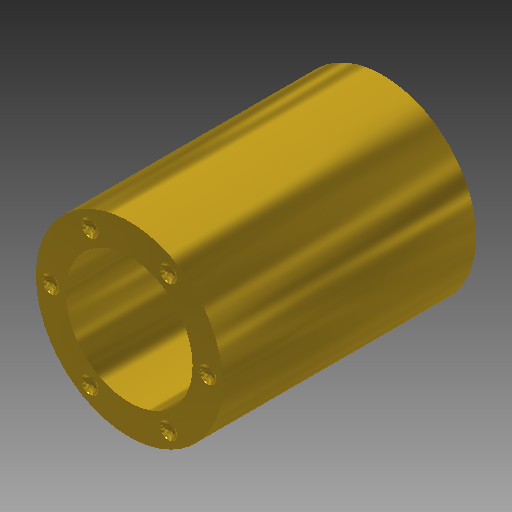
# Autodesk Inventor part: Electrode 1
Saved by Autodesk Inventor 2017 (Build 210142000, 142)
## iProperties
Created: 2009-05-06
Part Number: Electrode 1
Document SubType Name: Modeling
Designer: Serena
Material: Generic
Density: 1 g/cm^3
Appearance: Glossy - Gold
Author: Serena
Autodesk Inventor part; units mm, degrees
ref_plane "YZ Plane" through (0, 0, 0) normal (1, 0, 0) x (0, 1, 0)
ref_plane "XZ Plane" through (0, 0, 0) normal (0, 1, 0) x (-1, 0, 0)
ref_plane "XY Plane" through (0, 0, 0) normal (0, 0, 1) x (1, 0, 0)
sketch "Sketch1" plane through (0, 0, 0) normal (0, 0, 1) x (1, 0, 0)
  circle A0 centre (0, 0) radius 6.35
  circle A1 centre (0, 0) radius 9.35
  dimension "d0" = 12.7
  dimension "d1" = 18.7
  constraints: 2 centre point, 1 coincident
  measures "d0" diameter of A0
  measures "d1" diameter of A1
extrude "Extrusion1" add sketch "Sketch1" along normal blind 25.4
sketch "Sketch2" plane through (0, 0, 0) normal (0, 1, 0) x (-1, 0, 0)
  line L0 (-9.35, 0) -> (9.35, 0)
  line L1 (-9.35, 25.4) -> (9.35, 25.4)
  line L2 (-9.35, 25.4) -> (9.35, 25.4)
  line L3 (-9.35, 0) -> (9.35, 0)
  line L4 (6.35, 0) -> (6.35, 25.4)
  line L5 (9.35, 0) -> (9.35, 25.4)
  line L6 (-9.35, 0) -> (-9.35, 25.4)
  line L7 (-6.35, 0) -> (-6.35, 25.4)
  line L8 (7.85, 25.4) -> (7.85, 0)
  line L9 (7.85, 23.328674) -> (6.35, 23.328674)
  line L10 (9.35, 22.247069) -> (7.85, 22.247069)
  line L11 (12.106354, 26.15) -> (-10.018865, 26.15)
  line L12 (7.85, 25.4) -> (7.85, 27.239853)
  circle A0 centre (7.85, 26.15) radius 1
  line L13 (8.511438, 25.4) -> (7.188562, 25.4)
  line L14 (7.85, 25.4) -> (7.188562, 25.4)
  line L15 (7.85, 25.4) -> (7.85, 25.15)
  arc A1 (7.188562, 25.4) -> (7.85, 25.15) centre (7.85, 26.15) ccw
  dimension "d4" = 2
  dimension "d5" = 1.5
  constraints: 16 end point, 11 point on line, 5 point on circle, 4 perpendicular, 2 centre point, 2 concentric, 2 parallel, 1 collinear
  measures "d4" diameter of A0
  measures "d5" diameter of L1 L11
sketch "Sketch4" plane through (0, 0, 0) normal (0, 1, 0) x (-1, 0, 0)
  line L0 (9.35, 0) -> (9.35, 25.4)
  line L1 (6.35, 0) -> (6.35, 25.4)
  line L2 (-9.35, 25.4) -> (9.35, 25.4)
  line L3 (-9.35, 0) -> (9.35, 0)
  line L4 (7.85, 25.4) -> (7.85, 0)
  line L5 (9.35, 5.116219) -> (7.85, 5.116219)
  line L6 (7.85, 3.635363) -> (6.35, 3.635363)
  circle A0 centre (7.858912, -0.49996) radius 1
  line L7 (7.85, 0) -> (7.85, -2.207996)
  line L8 (7.85, 0) -> (7.85, 0.5)
  line L9 (7.85, 0) -> (6.992864, 0)
  arc A1 (7.85, 0.5) -> (6.992864, 0) centre (7.858912, -0.49996) ccw
  dimension "d11" = 2
  dimension "d12" = 0.5
  constraints: 12 end point, 8 point on line, 4 point on circle, 3 perpendicular, 2 centre point, 2 parallel, 1 concentric
  measures "d11" diameter of A0
  measures "d12" distance of L4.end L8.end
revolve "Revolution2" cut sketch "Sketch4" angle 360 about axis through (-7.85, 0, 25.4) along (0, 0, -1) picked at (7.319138, 0.055939) contours L3 A0 L4
pattern_circular "Circular Pattern1" count 6 over 360 about axis through (0, 0, 0) along (0, 0, 1) of "Revolution2"
sketch "Sketch5" plane through (0, 0, 0) normal (0, 1, 0) x (-1, 0, 0)
  line L0 (6.35, 0) -> (6.35, 25.4)
  line L1 (9.35, 0) -> (9.35, 25.4)
  line L2 (-9.35, 25.4) -> (9.35, 25.4)
  line L3 (-9.35, 0) -> (9.35, 0)
  line L4 (7.85, 25.4) -> (7.85, 0)
  line L5 (7.85, 23.017634) -> (9.35, 23.017634)
  line L6 (7.85, 21.744974) -> (6.35, 21.744974)
  line L7 (7.85, 25.4) -> (7.85, 28.066425)
  circle A0 centre (7.85, 25.9) radius 1
  line L8 (8.716025, 25.4) -> (6.983975, 25.4)
  line L9 (7.85, 25.4) -> (7.85, 24.9)
  arc A1 (6.983975, 25.4) -> (7.85, 24.9) centre (7.85, 25.9) ccw
  dimension "d17" = 2
  dimension "d18" = 0.5
  constraints: 12 end point, 10 point on line, 5 point on circle, 4 perpendicular, 2 centre point, 1 concentric, 1 parallel
  measures "d17" diameter of A0
  measures "d18" distance of L4.start L9.end
revolve "Revolution3" cut sketch "Sketch5" angle 360 about axis through (-7.85, 0, 25.4) along (0, 0, -1) picked at (8.38639, 25.343623) contours L2 A0 L4
pattern_circular "Circular Pattern2" count 6 over 360 about axis through (0, 0, 0) along (0, 0, 1) of "Revolution3"
body "Solid1"
